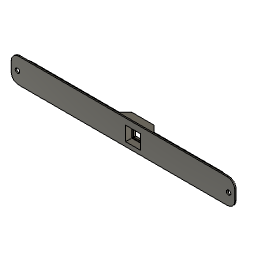
CoverUno (Autodesk Fusion 360 design; units mm, degrees)
Autodesk Fusion 360 part; units mm, degrees
sketch "Skizze1" plane through (0, 0, 0) normal (0, 1, 0) x (1, 0, 0)
  line L0 (0, 0) -> (164, 0)
  line L1 (164, 0) -> (164, -18)
  line L2 (164, -18) -> (0, -18)
  line L3 (0, -18) -> (0, 0)
  dimension "d1" = 18
  dimension "d2" = 164
  constraint horizontal L0
  constraint vertical L1
  constraint horizontal L2
  constraint vertical L3
  constraint coincident L0.start L3.end
  measures "d1" distance of L0.start L2.end
  measures "d2" distance of L1.end L2.end
extrude "Extrusion1" add sketch "Skizze1" along normal blind 8
fillet "Abrundung1" radius 5 4 edges at (0, 4, 18) (164, 4, 18) (0, 4, 0) (164, 4, 0)
sketch "Skizze2" plane through (0, 0, 0) normal (0, 1, 0) x (1, 0, 0)
  line L0 (-8, -19.5) -> (172, -19.5)
  line L1 (172, -19.5) -> (172, 0.5)
  line L2 (172, 0.5) -> (-8, 0.5)
  line L3 (-8, 0.5) -> (-8, -19.5)
  line L4 (-8, -9) -> (172, -9) construction
  circle A0 centre (-3, -9) radius 1.75
  circle A1 centre (167, -9) radius 1.75
  point P0 (0, -13)
  point P1 (164, -13)
  dimension "d7" = 0.5
  dimension "d8" = 19.5
  dimension "d9" = 9
  dimension "d10" = 3
  dimension "d11" = 3
  dimension "d12" = 3.5
  dimension "d13" = 5
  dimension "d14" = 5
  constraint horizontal L0
  constraint vertical L1
  constraint horizontal L2
  constraint vertical L3
  constraint coincident L3 L4.start
  constraint coincident L1 L4.end
  constraint perpendicular L1 L4
  constraint coincident L4 A0.centre
  constraint coincident L4 A1.centre
  constraint equal A0 A1
  measures "d7" vertical distance of origin L2.end
  measures "d8" vertical distance of origin L0.start
  measures "d9" vertical distance of origin L4.start
  measures "d10" horizontal distance of A0.centre P0
  measures "d11" horizontal distance of A1.centre P1
  measures "d12" diameter of A0
  measures "d13" horizontal distance of L0.start A0.centre
  measures "d14" distance of L4.end A1.centre
extrude "Extrusion2" add sketch "Skizze2" against normal blind 1
fillet "Abrundung2" radius 6 4 edges at (172, -0.5, 19.5) (172, -0.5, -0.5) (-8, -0.5, 19.5) (-8, -0.5, -0.5)
extrude "Extrusion3" cut 1 faces at (56.3333, 8, 12) along direction (0, -1, 0) blind 6
sketch "Skizze3" plane through (0, 2, 0) normal (0, 1, 0) x (-1, 0, 0)
  arc A0 (-164, 5) -> (-159, 0) centre (-159, 5) ccw
  line L0 (-159, 0) -> (-5, 0)
  arc A1 (-5, 0) -> (0, 5) centre (-5, 5) ccw
  line L1 (0, 5) -> (0, 13)
  arc A2 (0, 13) -> (-5, 18) centre (-5, 13) ccw
  line L2 (-5, 18) -> (-159, 18)
  arc A3 (-159, 18) -> (-164, 13) centre (-159, 13) ccw
  line L3 (-164, 13) -> (-164, 5)
  line L4 (-96, 14.5) -> (-84, 14.5)
  line L5 (-84, 14.5) -> (-84, 3)
  line L6 (-84, 3) -> (-96, 3)
  line L7 (-96, 3) -> (-96, 14.5)
  dimension "d21" = 68
  dimension "d22" = 3
  dimension "d23" = 3.5
  dimension "d24" = 12
  constraint horizontal L4
  constraint vertical L5
  constraint horizontal L6
  constraint vertical L7
  measures "d21" horizontal distance of A3.end L4.start
  measures "d22" vertical distance of A0.end L6.end
  measures "d23" vertical distance of L2.end L4.start
  measures "d24" distance of L4.start L4.end
extrude "Extrusion4" add sketch "Skizze3" along normal blind 3 contours L4 L5 L6 L7
sketch "Skizze4" plane through (0, 2, 0) normal (0, 1, 0) x (-1, 0, 0)
  line L0 (-96, 3) -> (-96, 14.5)
  line L1 (-96, 14.5) -> (-84, 14.5)
  line L2 (-84, 14.5) -> (-84, 3)
  line L3 (-84, 3) -> (-96, 3)
  arc A0 (-164, 5) -> (-159, 0) centre (-159, 5) ccw
  line L4 (-159, 0) -> (-5, 0)
  arc A1 (-5, 0) -> (0, 5) centre (-5, 5) ccw
  line L5 (0, 5) -> (0, 13)
  arc A2 (0, 13) -> (-5, 18) centre (-5, 13) ccw
  line L6 (-5, 18) -> (-159, 18)
  arc A3 (-159, 18) -> (-164, 13) centre (-159, 13) ccw
  line L7 (-164, 13) -> (-164, 5)
  line L8 (-99, 18) -> (-81, 18)
  line L9 (-81, 18) -> (-81, 0)
  line L10 (-81, 0) -> (-99, 0)
  line L11 (-99, 0) -> (-99, 18)
  dimension "d27" = 3.5
  dimension "d28" = 3
  dimension "d29" = 3
  dimension "d30" = 3
  constraint horizontal L8
  constraint vertical L9
  constraint horizontal L10
  constraint vertical L11
  measures "d27" vertical distance of L0.end L8.start
  measures "d28" vertical distance of L0.start L10.end
  measures "d29" horizontal distance of L0.end L8.start
  measures "d30" horizontal distance of L1.end L8.end
extrude "Extrusion5" add sketch "Skizze4" along normal blind 5 contours L4 L6 L8 L9 L10 L11
sketch "Skizze5" plane through (0, 5, 0) normal (0, 1, 0) x (-1, 0, 0)
  line L0 (-96, 3) -> (-84, 3)
  line L1 (-84, 3) -> (-84, 14.5)
  line L2 (-84, 14.5) -> (-96, 14.5)
  line L3 (-96, 14.5) -> (-96, 3)
  line L4 (-95.5, 14) -> (-84.5, 14)
  line L5 (-84.5, 14) -> (-84.5, 3.5)
  line L6 (-84.5, 3.5) -> (-95.5, 3.5)
  line L7 (-95.5, 3.5) -> (-95.5, 14)
  dimension "d33" = 0.5
  dimension "d34" = 0.5
  dimension "d35" = 0.5
  dimension "d36" = 0.5
  constraint horizontal L4
  constraint vertical L5
  constraint horizontal L6
  constraint vertical L7
  measures "d33" vertical distance of L2.end L4.start
  measures "d34" horizontal distance of L1.end L4.end
  measures "d35" horizontal distance of L2.end L4.start
  measures "d36" vertical distance of L0.start L6.end
extrude "Extrusion6" cut sketch "Skizze5" against normal blind 13 contours L4 L5 L6 L7
sketch "Skizze6" plane through (0, -1, 0) normal (0, -1, 0) x (1, 0, 0)
  line L0 (84.5, 3.5) -> (84.5, 14)
  line L1 (84.5, 14) -> (95.5, 14)
  line L2 (95.5, 14) -> (95.5, 3.5)
  line L3 (95.5, 3.5) -> (84.5, 3.5)
  arc A0 (-8, 5.5) -> (-2, -0.5) centre (-2, 5.5) ccw
  line L4 (-2, -0.5) -> (166, -0.5)
  arc A1 (166, -0.5) -> (172, 5.5) centre (166, 5.5) ccw
  line L5 (172, 5.5) -> (172, 13.5)
  arc A2 (172, 13.5) -> (166, 19.5) centre (166, 13.5) ccw
  line L6 (166, 19.5) -> (-2, 19.5)
  arc A3 (-2, 19.5) -> (-8, 13.5) centre (-2, 13.5) ccw
  line L7 (-8, 13.5) -> (-8, 5.5)
  circle A4 centre (-3, 9) radius 1.75
  circle A5 centre (167, 9) radius 1.75
  line L8 (84, 14.5) -> (96, 14.5)
  line L9 (96, 14.5) -> (96, 3)
  line L10 (96, 3) -> (84, 3)
  line L11 (84, 3) -> (84, 14.5)
  dimension "d39" = 0.5
  dimension "d40" = 0.5
  dimension "d41" = 0.5
  dimension "d42" = 0.5
  constraint horizontal L8
  constraint vertical L9
  constraint horizontal L10
  constraint vertical L11
  measures "d39" horizontal distance of L0.end L8.start
  measures "d40" horizontal distance of L1.end L8.end
  measures "d41" vertical distance of L2.end L9.end
  measures "d42" vertical distance of L0.end L8.start
extrude "Extrusion7" cut sketch "Skizze6" against normal blind 5 contours L8 L9 L10 L11
chamfer "Fase1" distance 5 angle 45 2 edges at (99, 2, 9) (81, 2, 9)
